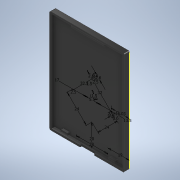
# Autodesk Inventor part: Top
Saved by Autodesk Inventor 2020 (Build 240168000, 168)
## iProperties
Created: 2021-06-19
Part Number: Top
Material: Generic
Document SubType Name: Modeling
Designer: micup
Density: 1 g/cm^3
Appearance: Glossy - Black
Author: micup
Autodesk Inventor part; units mm, degrees
ref_plane "YZ Plane" through (0, 0, 0) normal (1, 0, 0) x (0, 1, 0)
ref_plane "XZ Plane" through (0, 0, 0) normal (0, 1, 0) x (-1, 0, 0)
ref_plane "XY Plane" through (0, 0, 0) normal (0, 0, 1) x (1, 0, 0)
sketch "Sketch2" plane through (0, 0, 0) normal (0, 0, 1) x (1, 0, 0)
  line L0 (0, 0) -> (66, 0)
  line L1 (66, 0) -> (66, 91)
  line L2 (66, 91) -> (0, 91)
  line L3 (0, 91) -> (0, 0)
  line L4 (1.5, 1.5) -> (64.5, 1.5)
  line L5 (64.5, 1.5) -> (64.5, 89.5)
  line L6 (64.5, 89.5) -> (1.5, 89.5)
  line L7 (1.5, 89.5) -> (1.5, 1.5)
  line L8 (10.5, 80.5) -> (55.5, 80.5) construction
  line L9 (55.5, 80.5) -> (55.5, 10.5) construction
  line L10 (55.5, 10.5) -> (10.5, 10.5) construction
  line L11 (10.5, 10.5) -> (10.5, 80.5) construction
  line L12 (27, 0) -> (39, 0)
  line L13 (39, 0) -> (39, 1.5)
  line L14 (39, 1.5) -> (27, 1.5)
  line L15 (27, 1.5) -> (27, 0)
  line L16 (1, 1) -> (65, 1)
  line L17 (65, 1) -> (65, 90)
  line L18 (65, 90) -> (1, 90)
  line L19 (1, 90) -> (1, 1)
  line L20 (9, 1) -> (15, 1)
  line L21 (15, 1) -> (15, 0.6)
  line L22 (15, 0.6) -> (9, 0.6)
  line L23 (9, 0.6) -> (9, 1)
  line L24 (57, 0.6) -> (51, 0.6)
  line L25 (57, 1) -> (57, 0.6)
  line L26 (51, 0.6) -> (51, 1)
  line L27 (51, 1) -> (57, 1)
  line L28 (18, 90) -> (48, 90)
  line L29 (48, 90) -> (48, 90.5)
  line L30 (48, 90.5) -> (18, 90.5)
  line L31 (18, 90.5) -> (18, 90)
  line L32 (56.75, 4.1) -> (51.25, 4.1)
  line L33 (51, 3.85) -> (51, 2.6)
  line L34 (51, 2.6) -> (57, 2.6)
  line L35 (57, 2.6) -> (57, 3.85)
  line L36 (57, 2.6) -> (51, 2.6)
  line L37 (51, 2.6) -> (51, 2.45)
  line L38 (51.25, 2.2) -> (56.75, 2.2)
  line L39 (57, 2.45) -> (57, 2.6)
  arc A0 (57, 3.85) -> (56.75, 4.1) centre (56.75, 3.85) ccw
  arc A1 (51.25, 4.1) -> (51, 3.85) centre (51.25, 3.85) ccw
  arc A2 (51, 2.45) -> (51.25, 2.2) centre (51.25, 2.45) ccw
  arc A3 (56.75, 2.2) -> (57, 2.45) centre (56.75, 2.45) ccw
  line L40 (14.75, 4.1) -> (9.25, 4.1)
  line L41 (15, 2.6) -> (15, 3.85)
  arc A4 (15, 3.85) -> (14.75, 4.1) centre (14.75, 3.85) ccw
  arc A5 (14.75, 2.2) -> (15, 2.45) centre (14.75, 2.45) ccw
  line L42 (9, 2.6) -> (15, 2.6)
  line L43 (15, 2.45) -> (15, 2.6)
  line L44 (9.25, 2.2) -> (14.75, 2.2)
  arc A6 (9, 2.45) -> (9.25, 2.2) centre (9.25, 2.45) ccw
  line L45 (9, 3.85) -> (9, 2.6)
  arc A7 (9.25, 4.1) -> (9, 3.85) centre (9.25, 3.85) ccw
  line L46 (9, 2.6) -> (9, 2.45)
  line L47 (48, 88.4) -> (18, 88.4)
  line L48 (18, 88.4) -> (18, 87.15)
  line L49 (18.25, 86.9) -> (47.75, 86.9)
  line L50 (48, 87.15) -> (48, 88.4)
  line L51 (48, 88.4) -> (18, 88.4)
  line L52 (18, 88.4) -> (18, 88.55)
  line L53 (18.25, 88.8) -> (47.75, 88.8)
  line L54 (48, 88.55) -> (48, 88.4)
  arc A8 (18.25, 88.8) -> (18, 88.55) centre (18.25, 88.55) ccw
  arc A9 (18, 87.15) -> (18.25, 86.9) centre (18.25, 87.15) ccw
  arc A10 (47.75, 86.9) -> (48, 87.15) centre (47.75, 87.15) ccw
  arc A11 (48, 88.55) -> (47.75, 88.8) centre (47.75, 88.55) ccw
  point P0 (56.5, 81.5)
  point P1 (18, 88.8)
  dimension "d12" = 1.5
  dimension "d13" = 1.5
  dimension "d14" = 1.5
  dimension "d15" = 1.5
  dimension "d16" = 70
  dimension "d17" = 45
  dimension "d18" = 9
  dimension "d19" = 63
  dimension "d20" = 88
  dimension "d21" = 9
  dimension "d39" = 12
  dimension "d40" = 27
  dimension "d41" = 1
  dimension "d42" = 1
  dimension "d43" = 1
  dimension "d44" = 1
  dimension "d45" = 0.4
  dimension "d46" = 6
  dimension "d47" = 9
  dimension "d48" = 42
  dimension "d52" = 0.5
  dimension "d53" = 30
  dimension "d54" = 17
  dimension "d68" = 1.1
  dimension "d69" = 1.5
  dimension "d70" = 0.4
  dimension "d71" = 0.25
  dimension "d74" = 42
  dimension "d79" = 1.1
  dimension "d80" = 0.4
  dimension "d81" = 1.5
  dimension "d82" = 0.25
  constraints: 110 end point, 24 point on circle, 22 parallel, 16 tangent, 13 horizontal, 12 centre point, 11 perpendicular, 7 point on line, 6 equal radius, 1 collinear, 33 other
  measures "d12" distance between parallel lines of L2 L6
  measures "d13" distance between parallel lines of L0 L4
  measures "d14" distance between parallel lines of L1 L5
  measures "d15" distance between parallel lines of L3 L7
  measures "d16" distance between parallel lines of L10 L8
  measures "d17" distance between parallel lines of L9 L11
  measures "d18" distance between parallel lines of L7 L11
  measures "d19" distance between parallel lines of L5 L7
  measures "d20" distance between parallel lines of L4 L6
  measures "d21" distance between parallel lines of L6 L8
  measures "d39" distance between parallel lines of L13 L15
  measures "d40" distance between parallel lines of L3 L15
  measures "d41" distance between parallel lines of L2 L18
  measures "d42" distance between parallel lines of L1 L17
  measures "d43" distance between parallel lines of L3 L19
  measures "d44" distance between parallel lines of L0 L16
  measures "d45" distance between parallel lines of L16 L22
  measures "d46" distance between parallel lines of L21 L23
  measures "d47" distance between parallel lines of L23 L3
  measures "d48" distance of L22.start L24.start
  measures "d52" distance between parallel lines of L28 L30
  measures "d53" distance of L29.end L30.end
  measures "d54" distance from line of L19 L30.end
  measures "d68" distance between parallel lines of L4 L34
  measures "d69" distance between parallel lines of L34 L32
  measures "d70" distance between parallel lines of L34 L38
  measures "d71" radius of A0
  measures "d74" distance of L32.start L40.start
  measures "d79" distance between parallel lines of L6 L47
  measures "d80" distance between parallel lines of L53 L47
  measures "d81" distance between parallel lines of L49 L47
  measures "d82" radius of A8
extrude "Extrusion1" add sketch "Sketch2" along normal blind 1.5 contours L4 L7 L6 L5 | A0 L35 L34 L33 A1 L32 | L39 A3 L38 A2 L37 L34 | A4 L41 L42 L45 A7 L40 | L43 A5 L44 A6 L46 L42 | L50 A10 L49 A9 L48 L47 | L47 L52 A8 L53 A11 L54
extrude "Extrusion2" add sketch "Sketch2" along normal blind 4.5 contours L3 L2 L1 L0 L13 L16 L26 L24 L25 L17 L18 L29 L30 L31 L19 L23 L22 L21 L15 | L16 L19 L18 L17 L13 L4 L5 L6 L7 L15
extrude "Extrusion3" add sketch "Sketch2" along normal blind 4.5 contours L31 L30 L29 L18
extrude "Extrusion4" add sketch "Sketch2" along normal blind 4.5 contours L21 L22 L23 L16 | L16 L25 L24 L26
extrude "Extrusion7" add sketch "Sketch2" along normal blind 3 contours L15 L16 L13 L0 | L15 L4 L13 L16
sketch "Sketch3" plane through (0, 0, 1.5) normal (0, 0, 1) x (1, 0, 0)
  line L0 (0, 0) -> (63, 0)
  line L1 (63, 0) -> (63, 88)
  line L2 (63, 88) -> (0, 88)
  line L3 (0, 88) -> (0, 0)
  line L4 (1.5, 1.5) -> (61.5, 1.5)
  line L5 (61.5, 1.5) -> (61.5, 86.5)
  line L6 (61.5, 86.5) -> (1.5, 86.5)
  line L7 (1.5, 86.5) -> (1.5, 1.5)
  line L8 (9, 79) -> (54, 79) construction
  line L9 (54, 79) -> (54, 9) construction
  line L10 (54, 9) -> (9, 9) construction
  line L11 (9, 9) -> (9, 79) construction
  circle A0 centre (18.985, 69.431) radius 1.4
  circle A1 centre (44.015, 69.431) radius 1.4
  circle A2 centre (15.341, 31.556) radius 1.4
  circle A3 centre (47.659, 31.556) radius 1.4
  circle A4 centre (6.5, 81.5) radius 3
  circle A5 centre (56.5, 81.5) radius 3
  circle A6 centre (6.5, 6.5) radius 3
  circle A7 centre (56.5, 6.5) radius 3
  line L12 (25.5, 0) -> (37.5, 0)
  line L13 (37.5, 0) -> (37.5, 1.5)
  line L14 (37.5, 1.5) -> (25.5, 1.5)
  line L15 (25.5, 1.5) -> (25.5, 0)
  line L16 (1, 1) -> (62, 1)
  line L17 (62, 1) -> (62, 87)
  line L18 (62, 87) -> (1, 87)
  line L19 (1, 87) -> (1, 1)
  line L20 (7.5, 1) -> (13.5, 1)
  line L21 (13.5, 1) -> (13.5, 0.6)
  line L22 (13.5, 0.6) -> (7.5, 0.6)
  line L23 (7.5, 0.6) -> (7.5, 1)
  line L24 (55.5, 0.6) -> (49.5, 0.6)
  line L25 (55.5, 1) -> (55.5, 0.6)
  line L26 (49.5, 0.6) -> (49.5, 1)
  line L27 (49.5, 1) -> (55.5, 1)
  dimension "d101" = 1.5
  dimension "d102" = 1.5
  dimension "d103" = 1.5
  dimension "d104" = 1.5
  dimension "d105" = 70
  dimension "d106" = 45
  dimension "d107" = 7.5
  dimension "d108" = 60
  dimension "d109" = 85
  dimension "d110" = 7.5
  dimension "d111" = 2.8
  dimension "d112" = 2.8
  dimension "d113" = 2.8
  dimension "d114" = 2.8
  dimension "d115" = 6
  dimension "d116" = 6.341
  dimension "d117" = 6.341
  dimension "d118" = 9.985
  dimension "d119" = 9.985
  dimension "d120" = 22.556
  dimension "d121" = 22.556
  dimension "d122" = 9.569
  dimension "d123" = 9.569
  dimension "d124" = 5
  dimension "d125" = 5
  dimension "d126" = 50
  dimension "d127" = 75
  dimension "d128" = 12
  dimension "d129" = 25.5
  dimension "d130" = 1
  dimension "d131" = 1
  dimension "d132" = 1
  dimension "d133" = 1
  dimension "d134" = 0.4
  dimension "d135" = 6
  dimension "d136" = 7.5
  dimension "d137" = 42
  constraints: 56 end point, 12 parallel, 8 centre point, 8 horizontal, 6 perpendicular, 3 point on line, 1 vertical, 14 other
  measures "d101" distance between parallel lines of L2 L6
  measures "d102" distance between parallel lines of L0 L4
  measures "d103" distance between parallel lines of L1 L5
  measures "d104" distance between parallel lines of L3 L7
  measures "d105" distance between parallel lines of L10 L8
  measures "d106" distance between parallel lines of L9 L11
  measures "d107" distance between parallel lines of L7 L11
  measures "d108" distance between parallel lines of L5 L7
  measures "d109" distance between parallel lines of L4 L6
  measures "d110" distance between parallel lines of L6 L8
  measures "d111" diameter of A2
  measures "d112" diameter of A3
  measures "d113" diameter of A0
  measures "d114" diameter of A1
  measures "d115" diameter of A4
  measures "d116" distance from line of L11 A2.centre
  measures "d117" distance from line of L9 A3.centre
  measures "d118" distance from line of L11 A0.centre
  measures "d119" distance from line of L9 A1.centre
  measures "d120" distance from line of L10 A2.centre
  measures "d121" distance from line of L10 A3.centre
  measures "d122" distance from line of L8 A0.centre
  measures "d123" distance from line of L8 A1.centre
  measures "d124" distance from line of L6 A4.centre
  measures "d125" distance from line of L7 A4.centre
  measures "d126" distance of A4.centre A5.centre
  measures "d127" distance of A4.centre A6.centre
  measures "d128" distance between parallel lines of L13 L15
  measures "d129" distance between parallel lines of L3 L15
  measures "d130" distance between parallel lines of L2 L18
  measures "d131" distance between parallel lines of L1 L17
  measures "d132" distance between parallel lines of L3 L19
  measures "d133" distance between parallel lines of L0 L16
  measures "d134" distance between parallel lines of L16 L22
  measures "d135" distance between parallel lines of L21 L23
  measures "d136" distance between parallel lines of L23 L3
  measures "d137" distance of L22.start L25.end
extrude "Extrusion8" add sketch "Sketch2" along normal blind 3.5 contours L50 A10 L49 A9 L48 L47
sketch "Sketch4" plane through (18, 88.4, 1.5) normal (0, 1, 0) x (1, 0, 0)
  line L0 (30, -2) -> (0, -2) projected
  line L1 (30, 0) -> (30, -2) projected
  line L2 (0, -2) -> (30, -2)
  line L3 (30, -2) -> (30, -1.6)
  line L4 (30, -1.6) -> (0, -1.6)
  line L5 (0, -1.6) -> (0, -2)
  point P0 (-18, 1.5)
  dimension "d143" = 0.4
  constraints: 8 end point, 2 parallel, 1 horizontal, 1 perpendicular, 1 point on line
  measures "d143" distance between parallel lines of L0 L4
extrude "Extrusion9" add sketch "Sketch4" along normal blind 0.4
fillet "Fillet1" radius 0.5 1 edges at (33, 88.8, 3.5)
extrude "Extrusion10" add sketch "Sketch2" along normal blind 3.5 contours A0 L35 L34 L33 A1 L32 | A4 L41 L42 L45 A7 L40
sketch "Sketch5" plane through (51, 2.6, 1.5) normal (0, -1, 0) x (1, 0, 0)
  line L0 (-42, 0) -> (-42, 2) projected
  line L1 (-36, 0) -> (-36, 2) projected
  line L2 (-42, 2) -> (-36, 2)
  line L3 (-36, 2) -> (-36, 1.6)
  line L4 (-36, 1.6) -> (-42, 1.6)
  line L5 (-42, 1.6) -> (-42, 2)
  line L6 (6, 0) -> (6, 2) projected
  line L7 (0, 2) -> (6, 2)
  line L8 (6, 2) -> (6, 1.6)
  line L9 (6, 1.6) -> (0, 1.6)
  line L10 (0, 1.6) -> (0, 2)
  point P0 (-51, -1.5)
  dimension "d149" = 0.4
  dimension "d150" = 0.4
  constraints: 16 end point, 4 parallel, 2 horizontal, 2 perpendicular, 2 point on line
  measures "d149" distance between parallel lines of L2 L4
  measures "d150" distance between parallel lines of L7 L9
extrude "Extrusion11" add sketch "Sketch5" along normal blind 0.4
fillet "Fillet2" radius 0.5 2 edges at (12, 2.2, 3.5) (54, 2.2, 3.5)
fillet "Fillet3" radius 1 6 edges at (66, 0, 2.25) (0, 0, 2.25) (66, 91, 2.25) (0, 91, 2.25) (27, 0.75, 4.5) (39, 0.75, 4.5)
sketch "Sketch6" plane through (0, 0, 0) normal (0, 0, -1) x (-1, 0, 0)
  line L0 (-32.9999, 20) -> (-16.0294, 36.9706)
  line L1 (-16.0294, 36.9706) -> (-32.9999, 53.9411)
  line L2 (-32.9999, 53.9411) -> (-49.9705, 36.9706)
  line L3 (-49.9705, 36.9706) -> (-32.9999, 20)
  line L4 (-66, 1) -> (-66, 90) projected
  line L5 (0, 90) -> (0, 1) projected
  line L6 (-1, 0) -> (-65, 0) projected
  line L7 (-32.9999, 53.9411) -> (-38.7706, 59.7118) construction
  line L8 (-49.9705, 36.9706) -> (-59.2717, 46.2717) construction
  line L9 (-16.0294, 36.9706) -> (-3.6834, 24.6246) construction
  line L10 (-32.9999, 20) -> (-21.6281, 8.6281) construction
  line L11 (-35.192, 55.2846) -> (-37.6668, 57.7595)
  line L12 (-37.6668, 57.7595) -> (-39.0811, 56.3453)
  line L13 (-39.0811, 56.3453) -> (-36.6062, 53.8704)
  line L14 (-36.6062, 53.8704) -> (-35.192, 55.2846)
  line L15 (-39.5053, 55.921) -> (-40.9195, 54.5068)
  line L16 (-40.9195, 54.5068) -> (-38.4447, 52.0319)
  line L17 (-37.0304, 53.4462) -> (-39.5053, 55.921)
  line L18 (-38.4447, 52.0319) -> (-37.0304, 53.4462)
  line L19 (-41.3438, 54.0825) -> (-42.758, 52.6683)
  line L20 (-42.758, 52.6683) -> (-40.2831, 50.1935)
  line L21 (-38.8689, 51.6077) -> (-41.3438, 54.0825)
  line L22 (-40.2831, 50.1935) -> (-38.8689, 51.6077)
  line L23 (-43.1823, 52.2441) -> (-44.5965, 50.8299)
  line L24 (-44.5965, 50.8299) -> (-42.1216, 48.355)
  line L25 (-40.7074, 49.7692) -> (-43.1823, 52.2441)
  line L26 (-42.1216, 48.355) -> (-40.7074, 49.7692)
  line L27 (-45.0208, 50.4056) -> (-46.435, 48.9914)
  line L28 (-46.435, 48.9914) -> (-43.9601, 46.5165)
  line L29 (-42.5459, 47.9307) -> (-45.0208, 50.4056)
  line L30 (-43.9601, 46.5165) -> (-42.5459, 47.9307)
  line L31 (-46.8592, 48.5671) -> (-48.2734, 47.1529)
  line L32 (-48.2734, 47.1529) -> (-45.7986, 44.678)
  line L33 (-44.3844, 46.0922) -> (-46.8592, 48.5671)
  line L34 (-45.7986, 44.678) -> (-44.3844, 46.0922)
  line L35 (-48.6977, 46.7286) -> (-50.1119, 45.3144)
  line L36 (-50.1119, 45.3144) -> (-47.637, 42.8395)
  line L37 (-46.2228, 44.2538) -> (-48.6977, 46.7286)
  line L38 (-47.637, 42.8395) -> (-46.2228, 44.2538)
  line L39 (-50.5362, 44.8902) -> (-51.9504, 43.4759)
  line L40 (-51.9504, 43.4759) -> (-49.4755, 41.0011)
  line L41 (-48.0613, 42.4153) -> (-50.5362, 44.8902)
  line L42 (-49.4755, 41.0011) -> (-48.0613, 42.4153)
  line L43 (-52.3747, 43.0517) -> (-53.7889, 41.6375)
  line L44 (-53.7889, 41.6375) -> (-51.314, 39.1626)
  line L45 (-49.8998, 40.5768) -> (-52.3747, 43.0517)
  line L46 (-51.314, 39.1626) -> (-49.8998, 40.5768)
  line L47 (-14.6859, 34.7785) -> (-16.1001, 33.3643)
  line L48 (-16.1001, 33.3643) -> (-13.6252, 30.8894)
  line L49 (-12.211, 32.3037) -> (-14.6859, 34.7785)
  line L50 (-13.6252, 30.8894) -> (-12.211, 32.3037)
  line L51 (-16.5243, 32.9401) -> (-17.9386, 31.5258)
  line L52 (-17.9386, 31.5258) -> (-15.4637, 29.051)
  line L53 (-14.0495, 30.4652) -> (-16.5243, 32.9401)
  line L54 (-15.4637, 29.051) -> (-14.0495, 30.4652)
  line L55 (-18.3628, 31.1016) -> (-19.777, 29.6874)
  line L56 (-19.777, 29.6874) -> (-17.3022, 27.2125)
  line L57 (-15.888, 28.6267) -> (-18.3628, 31.1016)
  line L58 (-17.3022, 27.2125) -> (-15.888, 28.6267)
  line L59 (-20.2013, 29.2631) -> (-21.6155, 27.8489)
  line L60 (-21.6155, 27.8489) -> (-19.1406, 25.374)
  line L61 (-17.7264, 26.7882) -> (-20.2013, 29.2631)
  line L62 (-19.1406, 25.374) -> (-17.7264, 26.7882)
  line L63 (-22.0398, 27.4246) -> (-23.454, 26.0104)
  line L64 (-23.454, 26.0104) -> (-20.9791, 23.5355)
  line L65 (-19.5649, 24.9497) -> (-22.0398, 27.4246)
  line L66 (-20.9791, 23.5355) -> (-19.5649, 24.9497)
  line L67 (-23.8783, 25.5861) -> (-25.2925, 24.1719)
  line L68 (-25.2925, 24.1719) -> (-22.8176, 21.6971)
  line L69 (-21.4034, 23.1113) -> (-23.8783, 25.5861)
  line L70 (-22.8176, 21.6971) -> (-21.4034, 23.1113)
  line L71 (-25.7167, 23.7477) -> (-27.131, 22.3335)
  line L72 (-27.131, 22.3335) -> (-24.6561, 19.8586)
  line L73 (-23.2419, 21.2728) -> (-25.7167, 23.7477)
  line L74 (-24.6561, 19.8586) -> (-23.2419, 21.2728)
  line L75 (-27.5552, 21.9092) -> (-28.9694, 20.495)
  line L76 (-28.9694, 20.495) -> (-26.4946, 18.0201)
  line L77 (-25.0803, 19.4343) -> (-27.5552, 21.9092)
  line L78 (-26.4946, 18.0201) -> (-25.0803, 19.4343)
  line L79 (-29.3937, 20.0707) -> (-30.8079, 18.6565)
  line L80 (-30.8079, 18.6565) -> (-28.333, 16.1816)
  line L81 (-26.9188, 17.5958) -> (-29.3937, 20.0707)
  line L82 (-28.333, 16.1816) -> (-26.9188, 17.5958)
  line L83 (-51.314, 34.7785) -> (-53.4353, 32.6572)
  line L84 (-53.4353, 32.6572) -> (-52.0211, 31.243)
  line L85 (-52.0211, 31.243) -> (-49.8998, 33.3643)
  line L86 (-49.8998, 33.3643) -> (-51.314, 34.7785)
  line L87 (-49.9705, 36.9706) -> (-58.9154, 28.0257) construction
  line L88 (-32.9999, 20) -> (-40.9195, 12.0804) construction
  line L89 (-49.4755, 32.9401) -> (-51.5968, 30.8187)
  line L90 (-51.5968, 30.8187) -> (-50.1826, 29.4045)
  line L91 (-50.1826, 29.4045) -> (-48.0613, 31.5258)
  line L92 (-48.0613, 31.5258) -> (-49.4755, 32.9401)
  line L93 (-47.637, 31.1016) -> (-49.7584, 28.9803)
  line L94 (-49.7584, 28.9803) -> (-48.3442, 27.566)
  line L95 (-48.3442, 27.566) -> (-46.2228, 29.6874)
  line L96 (-46.2228, 29.6874) -> (-47.637, 31.1016)
  line L97 (-45.7986, 29.2631) -> (-47.9199, 27.1418)
  line L98 (-47.9199, 27.1418) -> (-46.5057, 25.7276)
  line L99 (-46.5057, 25.7276) -> (-44.3844, 27.8489)
  line L100 (-44.3844, 27.8489) -> (-45.7986, 29.2631)
  line L101 (-43.9601, 27.4246) -> (-46.0814, 25.3033)
  line L102 (-46.0814, 25.3033) -> (-44.6672, 23.8891)
  line L103 (-44.6672, 23.8891) -> (-42.5459, 26.0104)
  line L104 (-42.5459, 26.0104) -> (-43.9601, 27.4246)
  line L105 (-42.1216, 25.5861) -> (-44.2429, 23.4648)
  line L106 (-44.2429, 23.4648) -> (-42.8287, 22.0506)
  line L107 (-42.8287, 22.0506) -> (-40.7074, 24.1719)
  line L108 (-40.7074, 24.1719) -> (-42.1216, 25.5861)
  line L109 (-40.2831, 23.7477) -> (-42.4045, 21.6263)
  line L110 (-42.4045, 21.6263) -> (-40.9902, 20.2121)
  line L111 (-40.9902, 20.2121) -> (-38.8689, 22.3335)
  line L112 (-38.8689, 22.3335) -> (-40.2831, 23.7477)
  line L113 (-38.4447, 21.9092) -> (-40.566, 19.7879)
  line L114 (-40.566, 19.7879) -> (-39.1518, 18.3737)
  line L115 (-39.1518, 18.3737) -> (-37.0304, 20.495)
  line L116 (-37.0304, 20.495) -> (-38.4447, 21.9092)
  line L117 (-36.6062, 20.0707) -> (-38.7275, 17.9494)
  line L118 (-38.7275, 17.9494) -> (-37.3133, 16.5352)
  line L119 (-37.3133, 16.5352) -> (-35.192, 18.6565)
  line L120 (-35.192, 18.6565) -> (-36.6062, 20.0707)
  line L121 (-28.6866, 57.4059) -> (-30.8079, 55.2846)
  line L122 (-30.8079, 55.2846) -> (-29.3937, 53.8704)
  line L123 (-29.3937, 53.8704) -> (-27.2724, 55.9917)
  line L124 (-27.2724, 55.9917) -> (-28.6866, 57.4059)
  line L125 (-26.8481, 55.5675) -> (-28.9694, 53.4462)
  line L126 (-28.9694, 53.4462) -> (-27.5552, 52.0319)
  line L127 (-27.5552, 52.0319) -> (-25.4339, 54.1533)
  line L128 (-25.4339, 54.1533) -> (-26.8481, 55.5675)
  line L129 (-25.0096, 53.729) -> (-27.131, 51.6077)
  line L130 (-27.131, 51.6077) -> (-25.7167, 50.1935)
  line L131 (-25.7167, 50.1935) -> (-23.5954, 52.3148)
  line L132 (-23.5954, 52.3148) -> (-25.0096, 53.729)
  line L133 (-23.1712, 51.8905) -> (-25.2925, 49.7692)
  line L134 (-25.2925, 49.7692) -> (-23.8783, 48.355)
  line L135 (-23.8783, 48.355) -> (-21.7569, 50.4763)
  line L136 (-21.7569, 50.4763) -> (-23.1712, 51.8905)
  line L137 (-21.3327, 50.052) -> (-23.454, 47.9307)
  line L138 (-23.454, 47.9307) -> (-22.0398, 46.5165)
  line L139 (-22.0398, 46.5165) -> (-19.9185, 48.6378)
  line L140 (-19.9185, 48.6378) -> (-21.3327, 50.052)
  line L141 (-19.4942, 48.2136) -> (-21.6155, 46.0922)
  line L142 (-21.6155, 46.0922) -> (-20.2013, 44.678)
  line L143 (-20.2013, 44.678) -> (-18.08, 46.7993)
  line L144 (-18.08, 46.7993) -> (-19.4942, 48.2136)
  line L145 (-17.6557, 46.3751) -> (-19.777, 44.2538)
  line L146 (-19.777, 44.2538) -> (-18.3628, 42.8395)
  line L147 (-18.3628, 42.8395) -> (-16.2415, 44.9609)
  line L148 (-16.2415, 44.9609) -> (-17.6557, 46.3751)
  line L149 (-15.8172, 44.5366) -> (-17.9386, 42.4153)
  line L150 (-17.9386, 42.4153) -> (-16.5243, 41.0011)
  line L151 (-16.5243, 41.0011) -> (-14.403, 43.1224)
  line L152 (-14.403, 43.1224) -> (-15.8172, 44.5366)
  line L153 (-13.9788, 42.6981) -> (-16.1001, 40.5768)
  line L154 (-16.1001, 40.5768) -> (-14.6859, 39.1626)
  line L155 (-14.6859, 39.1626) -> (-12.5646, 41.2839)
  line L156 (-12.5646, 41.2839) -> (-13.9788, 42.6981)
  line L157 (-49.9705, 36.9706) -> (-16.0294, 36.9706) construction
  line L158 (-32.9999, 20) -> (-32.9999, 53.9411) construction
  circle A0 centre (-32.9999, 36.9706) radius 8.5
  circle A1 centre (-32.9999, 36.9706) radius 6.75
  line L159 (-35.3288, 44.3309) -> (-30.4618, 41.7692)
  line L160 (-35.3288, 44.3309) -> (-36.0274, 43.0035)
  line L161 (-36.0274, 43.0035) -> (-31.1604, 40.4418)
  line L162 (-31.1604, 40.4418) -> (-30.4618, 41.7692)
  line L163 (-47, 13.9467) -> (-19, 13.9467) construction
  line L164 (-19, 13.9467) -> (-19, 3.7834) construction
  line L165 (-19, 3.7834) -> (-47, 3.7834) construction
  line L166 (-47, 3.7834) -> (-47, 13.9467) construction
  line L167 (-31.6284, 48.3999) -> (-35.9861, 44.9287)
  line L168 (-31.6284, 48.3999) -> (-30.4638, 47.4098)
  line L169 (-30.4638, 47.4098) -> (-34.8216, 43.9386)
  line L170 (-34.8216, 43.9386) -> (-35.9861, 44.9287)
  spline S0 degree 2 poles (-38.3536, 8.8601) (-38.3536, 8.0049) (-39.1, 6.6604) (-39.6685, 6.2995) knots 0 0 0 1 2 2 2
  spline S1 degree 2 poles (-39.6685, 6.2995) (-40.143, 5.993) (-41.2602, 5.8151) (-41.888, 5.8151) knots 0 0 0 1 2 2 2
  line L171 (-41.888, 5.8151) -> (-43.7961, 5.8151)
  line L172 (-43.7961, 5.8151) -> (-43.7961, 11.9151)
  line L173 (-43.7961, 11.9151) -> (-41.9078, 11.9151)
  spline S2 degree 2 poles (-41.9078, 11.9151) (-41.2652, 11.9151) (-40.143, 11.7519) (-39.6487, 11.4356) knots 0 0 0 1 2 2 2
  spline S3 degree 2 poles (-39.6487, 11.4356) (-39.0506, 11.05) (-38.3536, 9.745) (-38.3536, 8.8601) knots 0 0 0 1 2 2 2
  spline S4 degree 2 poles (-39.9255, 8.87) (-39.9255, 9.4731) (-40.3408, 10.3332) (-40.7659, 10.5754) knots 0 0 0 1 2 2 2
  spline S5 degree 2 poles (-40.7659, 10.5754) (-41.0773, 10.7435) (-41.7595, 10.7781) (-42.234, 10.7781) knots 0 0 0 1 2 2 2
  line L174 (-42.234, 10.7781) -> (-42.2637, 10.7781)
  line L175 (-42.2637, 10.7781) -> (-42.2637, 6.957)
  line L176 (-42.2637, 6.957) -> (-42.234, 6.957)
  spline S6 degree 2 poles (-42.234, 6.957) (-41.7199, 6.957) (-41.013, 6.9916) (-40.6917, 7.1942) knots 0 0 0 1 2 2 2
  spline S7 degree 2 poles (-40.6917, 7.1942) (-40.316, 7.4315) (-39.9255, 8.2669) (-39.9255, 8.87) knots 0 0 0 1 2 2 2
  spline S8 degree 2 poles (-34.8142, 5.6964) (-36.1884, 5.6964) (-37.7999, 7.3574) (-37.7999, 8.8601) knots 0 0 0 1 2 2 2
  spline S9 degree 2 poles (-37.7999, 8.8601) (-37.7999, 10.3085) (-36.1835, 12.0337) (-34.8092, 12.0337) knots 0 0 0 1 2 2 2
  spline S10 degree 2 poles (-34.8092, 12.0337) (-34.4484, 12.0337) (-33.8651, 11.9497) (-33.5981, 11.8805) knots 0 0 0 1 2 2 2
  spline S11 degree 2 poles (-33.5981, 11.8805) (-33.3905, 11.8162) (-32.9011, 11.6036) (-32.7479, 11.5245) knots 0 0 0 1 2 2 2
  line L177 (-32.7479, 11.5245) -> (-32.7479, 10.0712)
  line L178 (-32.7479, 10.0712) -> (-32.9011, 10.0712)
  spline S12 degree 2 poles (-32.9011, 10.0712) (-33.0148, 10.1701) (-33.351, 10.4469) (-33.5635, 10.5754) knots 0 0 0 1 2 2 2
  spline S13 degree 2 poles (-33.5635, 10.5754) (-33.7761, 10.7089) (-34.2853, 10.8918) (-34.567, 10.8918) knots 0 0 0 1 2 2 2
  spline S14 degree 2 poles (-34.567, 10.8918) (-34.8982, 10.8918) (-35.4469, 10.6842) (-35.699, 10.4222) knots 0 0 0 1 2 2 2
  spline S15 degree 2 poles (-35.699, 10.4222) (-35.9264, 10.1899) (-36.2181, 9.394) (-36.2181, 8.8552) knots 0 0 0 1 2 2 2
  spline S16 degree 2 poles (-36.2181, 8.8552) (-36.2181, 8.2867) (-35.9165, 7.5106) (-35.6694, 7.2733) knots 0 0 0 1 2 2 2
  spline S17 degree 2 poles (-35.6694, 7.2733) (-35.4321, 7.041) (-34.8488, 6.8383) (-34.5571, 6.8383) knots 0 0 0 1 2 2 2
  spline S18 degree 2 poles (-34.5571, 6.8383) (-34.2556, 6.8383) (-33.7069, 7.041) (-33.519, 7.1646) knots 0 0 0 1 2 2 2
  spline S19 degree 2 poles (-33.519, 7.1646) (-33.3114, 7.2882) (-33, 7.5501) (-32.8863, 7.654) knots 0 0 0 1 2 2 2
  line L179 (-32.8863, 7.654) -> (-32.7479, 7.654)
  line L180 (-32.7479, 7.654) -> (-32.7479, 6.2204)
  spline S20 degree 2 poles (-32.7479, 6.2204) (-32.916, 6.1413) (-33.3559, 5.9436) (-33.5932, 5.8744) knots 0 0 0 1 2 2 2
  spline S21 degree 2 poles (-33.5932, 5.8744) (-33.8799, 5.7854) (-34.3792, 5.6964) (-34.8142, 5.6964) knots 0 0 0 1 2 2 2
  line L181 (-32.5007, 5.8151) -> (-30.4394, 11.9151)
  line L182 (-30.4394, 11.9151) -> (-28.7686, 11.9151)
  line L183 (-28.7686, 11.9151) -> (-26.7072, 5.8151)
  line L184 (-26.7072, 5.8151) -> (-28.2841, 5.8151)
  line L185 (-28.2841, 5.8151) -> (-28.6647, 7.0608)
  line L186 (-28.6647, 7.0608) -> (-30.5827, 7.0608)
  line L187 (-30.5827, 7.0608) -> (-30.9683, 5.8151)
  line L188 (-30.9683, 5.8151) -> (-32.5007, 5.8151)
  line L189 (-29.0009, 8.1681) -> (-29.6237, 10.1849)
  line L190 (-29.6237, 10.1849) -> (-30.2515, 8.1681)
  line L191 (-30.2515, 8.1681) -> (-29.0009, 8.1681)
  line L192 (-26.0992, 5.8151) -> (-26.0992, 11.9151)
  line L193 (-26.0992, 11.9151) -> (-21.9765, 11.9151)
  line L194 (-21.9765, 11.9151) -> (-21.9765, 10.7534)
  line L195 (-21.9765, 10.7534) -> (-24.5767, 10.7534)
  line L196 (-24.5767, 10.7534) -> (-24.5767, 9.6807)
  line L197 (-24.5767, 9.6807) -> (-22.1792, 9.6807)
  line L198 (-22.1792, 9.6807) -> (-22.1792, 8.519)
  line L199 (-22.1792, 8.519) -> (-24.5767, 8.519)
  line L200 (-24.5767, 8.519) -> (-24.5767, 6.9767)
  line L201 (-24.5767, 6.9767) -> (-21.9765, 6.9767)
  line L202 (-21.9765, 6.9767) -> (-21.9765, 5.8151)
  line L203 (-21.9765, 5.8151) -> (-26.0992, 5.8151)
  point P0 (0, 0)
  point P1 (-34.0215, 43.6428)
  point P2 (-32.8992, 45.47)
  dimension "d184" = 17
  dimension "d185" = 13.5
  dimension "d155" = 24
  dimension "d156" = 24
  dimension "d157" = 16.0295
  dimension "d159" = 20
  dimension "d160" = 2.5
  dimension "d161" = 0.6
  dimension "d162" = 2
  dimension "d165" = 2.6
  dimension "d168" = 32.5
  dimension "d171" = 2.5
  dimension "d172" = 2.5
  dimension "d173" = 0.6
  dimension "d174" = 2
  dimension "d177" = 2.6
  dimension "d180" = 32
  dimension "d183" = 2.5
  dimension "d192" = 1.5
  dimension "d194" = 5.5
  dimension "d199" = 28
  dimension "d200" = 19
  dimension "d205" = 1.5
  constraints: 328 end point, 9 parallel, 8 collinear, 7 perpendicular, 1 coincident, 1 horizontal alignment, 1 midpoint, 280 other
  measures "d155" distance between parallel lines of L0 L2
  measures "d156" distance between parallel lines of L1 L3
  measures "d157" distance from line of L4 L2.end
  measures "d159" distance from line of L6 L0.start
  measures "d160" distance between parallel lines of L2 L14
  measures "d161" distance between parallel lines of L7 L11
  measures "d162" distance between parallel lines of L11 L13
  measures "d165" distance of L11.end L15.start
  measures "d168" distance of L11.end L47.start
  measures "d171" distance between parallel lines of L47 L0
  measures "d172" distance between parallel lines of L3 L86
  measures "d173" distance between parallel lines of L87 L83
  measures "d174" distance between parallel lines of L85 L83
  measures "d177" distance of L83.start L89.start
  measures "d180" distance of L83.start L121.start
  measures "d183" distance between parallel lines of L122 L1
  measures "d192" distance between parallel lines of L159 L161
  measures "d194" distance between parallel lines of L162 L160
  measures "d199" distance between parallel lines of L164 L166
  measures "d200" distance between parallel lines of L4 L166
  measures "d205" distance between parallel lines of L169 L167
extrude "Extrusion12" add sketch "Sketch6" along normal blind 0.5 contours S0 S1 L171 L172 L173 S2 S3 | S8 S9 S10 S11 L177 L178 S12 S13 S14 S15 S16 S17 S18 S19 L179 L180 S20 S21 | L181 L182 L183 L184 L185 L186 L187 L188 | L192 L193 L194 L195 L196 L197 L198 L199 L200 L201 L202 L203
extrude "Extrusion14" add sketch "Sketch6" along normal blind 0.9 contours L3 L2 L1 L0 | A1 L161 L162 L159 picked at (-34.7313, 34.3278)
extrude "Extrusion15" add sketch "Sketch6" along normal blind 0.5 contours L170 L159 L160 A1 L169 A0 | L167 L168 L169 A0 | A0 L169 L159 L170 | L170 L169 L159 A1 L160 | L159 L169 L170 | L159 L162 L161 A1 | A1 L161 L162 L159
extrude "Extrusion16" add sketch "Sketch6" along normal blind 0.5 contours L14 L13 L12 L11 | L17 L18 L16 L15 | L21 L22 L20 L19 | L25 L26 L24 L23 | L29 L30 L28 L27 | L33 L34 L32 L31 | L37 L38 L36 L35 | L41 L42 L40 L39 | L45 L46 L44 L43 | L49 L50 L48 L47 | L53 L54 L52 L51 | L57 L58 L56 L55 | L61 L62 L60 L59 | L65 L66 L64 L63 | L69 L70 L68 L67 | L73 L74 L72 L71 | L77 L78 L76 L75 | L81 L82 L80 L79 | L86 L85 L84 L83 | L92 L91 L90 L89 | L96 L95 L94 L93 | L100 L99 L98 L97 | L104 L103 L102 L101 | L108 L107 L106 L105 | L112 L111 L110 L109 | L116 L115 L114 L113 | L120 L119 L118 L117 | L124 L123 L122 L121 | L128 L127 L126 L125 | L132 L131 L130 L129 | L136 L135 L134 L133 | L140 L139 L138 L137 | L144 L143 L142 L141 | L148 L147 L146 L145 | L152 L151 L150 L149 | L156 L155 L154 L153
body "Solid1"
